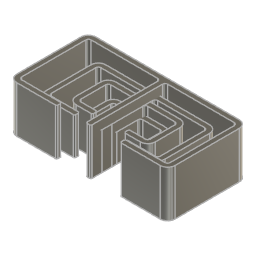
cable clip (Autodesk Fusion 360 design; units mm, degrees)
Autodesk Fusion 360 part; units mm, degrees
other "Base Mesh Feature1"
sketch "Sketch1" plane through (0, 0, 0) normal (0, 0, 1) x (1, 0, 0) in component "Clip-medium"
  line L0 (13, 8) -> (-13, 8)
  line L1 (-16, 5) -> (-16, -5)
  line L2 (16, -5) -> (16, 5)
  line L3 (16, 8) -> (-16, -8) construction
  line L4 (-16, 8) -> (16, -8) construction
  line L5 (-6.4, -8) -> (6.4, -8) construction
  line L6 (6.4, -8) -> (6.4, -6)
  line L7 (6.4, -6) -> (-6.4, -6) construction
  line L8 (-6.4, -6) -> (-6.4, -8)
  arc A0 (-13, 8) -> (-16, 5) centre (-13, 5) ccw
  arc A1 (16, 5) -> (13, 8) centre (13, 5) ccw
  arc A2 (13, -8) -> (16, -5) centre (13, -5) ccw
  arc A3 (-16, -5) -> (-13, -8) centre (-13, -5) ccw
  line L9 (-13, -8) -> (-6.4, -8)
  line L10 (6.4, -8) -> (13, -8)
  line L11 (6.4, -6) -> (13, -6)
  arc A4 (13, -6) -> (14, -5) centre (13, -5) ccw
  line L12 (14, -5) -> (14, 5)
  arc A5 (14, 5) -> (13, 6) centre (13, 5) ccw
  arc A6 (-13, 6) -> (-14, 5) centre (-13, 5) ccw
  line L13 (-14, 5) -> (-14, -5)
  arc A7 (-14, -5) -> (-13, -6) centre (-13, -5) ccw
  line L14 (-13, -6) -> (-6.4, -6)
  line L15 (0, 1.75) -> (0, 22.5) construction
  line L16 (-1, -8) -> (1, -8)
  line L17 (1, -8) -> (1, 6)
  line L18 (-1, 6) -> (-1, -8)
  line L19 (13, 6) -> (1, 6)
  line L20 (-1, 6) -> (-13, 6)
  dimension "d21" = 32
  dimension "d22" = 16
  dimension "d24" = 3
  dimension "d25" = 3
  dimension "d26" = 3
  dimension "d27" = 3
  dimension "d29" = 12.8
  dimension "d30" = 2
  constraint horizontal L0
  constraint perpendicular L0 L1
  constraint parallel L0 L9
  constraint parallel L1 L2
  constraint coincident L3 origin
  constraint coincident L4 origin
  constraint horizontal L5
  constraint vertical L6
  constraint horizontal L7
  constraint vertical L8
  constraint coincident L4.start L1
  constraint coincident L4.start L0
  constraint tangent L1 A0
  constraint tangent L0 A0
  constraint coincident L3.start L0
  constraint coincident L3.start L2
  constraint tangent L0 A1
  constraint tangent L2 A1
  constraint coincident L4.end L2
  constraint coincident L4.end L9
  constraint tangent L2 A2
  constraint tangent A2 L9
  constraint coincident L3.end L1
  constraint coincident L3.end L9
  constraint tangent L1 A3
  constraint tangent A3 L9
  constraint collinear L9 L10
  constraint horizontal L16
  constraint vertical L17
  constraint vertical L18
  constraint coincident L5 L16.start
  constraint concentric A2 A4
  constraint concentric A1 A5
  constraint concentric A0 A6
  constraint concentric A3 A7
  constraint tangent L13 A7
  constraint tangent A5 L19
  constraint tangent A4 L12
  constraint tangent L12 A5
  constraint tangent A6 L19
  constraint tangent A6 L13
  constraint collinear L19 L20
  constraint coincident L7.end L8.start
  measures "d21" distance of L3.end L4.end
  measures "d22" distance of L4.start L3.end
  measures "d24" radius of A0
  measures "d25" radius of A1
  measures "d26" radius of A2
  measures "d27" radius of A3
  measures "d29" distance of L7.end L6.end
  measures "d30" distance of L16.start L16.end
extrude "Extrude1" add sketch "Sketch1" along normal blind 15 makes body 1 in component "Clip-medium"
fillet "Fillet1" radius 0.5 6 edges at (-6.4, -8, 7.5) (-6.4, -6, 7.5) (-1, -8, 7.5) (1, -8, 7.5) (6.4, -8, 7.5) (6.4, -6, 7.5) on bodies 1 in component "Clip-medium"
fillet "Fillet1'" radius 1 2 edges at (-1, 6, 7.5) (1, 6, 7.5) on bodies 1 in component "Clip-medium"
sketch "Sketch1 (2)" plane through (0, 0, 0) normal (0, 0, 1) x (1, 0, 0) in component "Clip-small"
  line L0 (9, 6) -> (-9, 6)
  line L1 (-12, 3) -> (-12, -3)
  line L2 (12, -3) -> (12, 3)
  line L3 (12, 6) -> (-12, -6) construction
  line L4 (-12, 6) -> (12, -6) construction
  line L5 (-4.8, -6) -> (4.8, -6) construction
  line L6 (4.8, -6) -> (4.8, -4)
  line L7 (4.8, -4) -> (-4.8, -4) construction
  line L8 (-4.8, -4) -> (-4.8, -6)
  arc A0 (-9, 6) -> (-12, 3) centre (-9, 3) ccw
  arc A1 (12, 3) -> (9, 6) centre (9, 3) ccw
  arc A2 (9, -6) -> (12, -3) centre (9, -3) ccw
  arc A3 (-12, -3) -> (-9, -6) centre (-9, -3) ccw
  line L9 (-9, -6) -> (-4.8, -6)
  line L10 (4.8, -6) -> (9, -6)
  line L11 (4.8, -4) -> (9, -4)
  arc A4 (9, -4) -> (10, -3) centre (9, -3) ccw
  line L12 (10, -3) -> (10, 3)
  arc A5 (10, 3) -> (9, 4) centre (9, 3) ccw
  arc A6 (-9, 4) -> (-10, 3) centre (-9, 3) ccw
  line L13 (-10, 3) -> (-10, -3)
  arc A7 (-10, -3) -> (-9, -4) centre (-9, -3) ccw
  line L14 (-9, -4) -> (-4.8, -4)
  line L15 (0, 1.75) -> (0, 22.5) construction
  line L16 (-1.0119, -6) -> (0.9881, -6)
  line L17 (0.9881, -6) -> (0.9881, 4)
  line L18 (-1.0119, 4) -> (-1.0119, -6)
  line L19 (9, 4) -> (0.9881, 4)
  line L20 (-1.0119, 4) -> (-9, 4)
  dimension "d21_1" = 24
  dimension "d22_1" = 12
  dimension "d24_1" = 3
  dimension "d25_1" = 3
  dimension "d26_1" = 3
  dimension "d27_1" = 3
  dimension "d29_1" = 9.6
  dimension "d30_1" = 2
  constraint horizontal L0
  constraint perpendicular L0 L1
  constraint parallel L0 L9
  constraint parallel L1 L2
  constraint coincident L3 origin
  constraint coincident L4 origin
  constraint horizontal L5
  constraint vertical L6
  constraint horizontal L7
  constraint vertical L8
  constraint coincident L4.start L1
  constraint coincident L4.start L0
  constraint tangent L1 A0
  constraint tangent L0 A0
  constraint coincident L3.start L0
  constraint coincident L3.start L2
  constraint tangent L0 A1
  constraint tangent L2 A1
  constraint coincident L4.end L2
  constraint coincident L4.end L9
  constraint tangent L2 A2
  constraint tangent A2 L9
  constraint coincident L3.end L1
  constraint coincident L3.end L9
  constraint tangent L1 A3
  constraint tangent A3 L9
  constraint collinear L9 L10
  constraint horizontal L16
  constraint vertical L17
  constraint vertical L18
  constraint coincident L5 L16.start
  constraint concentric A2 A4
  constraint concentric A1 A5
  constraint concentric A0 A6
  constraint concentric A3 A7
  constraint tangent L13 A7
  constraint tangent A5 L19
  constraint tangent A4 L12
  constraint tangent L12 A5
  constraint tangent A6 L19
  constraint tangent A6 L13
  constraint collinear L19 L20
  constraint coincident L7.end L8.start
  measures "d21_1" distance of L3.end L4.end
  measures "d22_1" distance of L4.start L3.end
  measures "d24_1" radius of A0
  measures "d25_1" radius of A1
  measures "d26_1" radius of A2
  measures "d27_1" radius of A3
  measures "d29_1" distance of L7.end L6.end
  measures "d30_1" distance of L16.start L16.end
extrude "Extrude1'" add sketch "Sketch1 (2)" along normal blind 11.25 separate body makes body 2 in component "Clip-small"
fillet "Fillet1''" radius 0.5 6 edges at (-4.8, -6, 5.625) (-4.8, -4, 5.625) (-1.0119, -6, 5.625) (0.9881, -6, 5.625) (4.8, -6, 5.625) (4.8, -4, 5.625) on bodies 2 in component "Clip-small"
fillet "Fillet1'''" radius 1 2 edges at (-1.0119, 4, 5.625) (0.9881, 4, 5.625) on bodies 2 in component "Clip-small"
sketch "Sketch1 (3)" plane through (0, 0, 0) normal (0, 0, 1) x (1, 0, 0) in component "Clip-large"
  line L0 (21, 12) -> (-21, 12)
  line L1 (-24, 9) -> (-24, -9)
  line L2 (24, -9) -> (24, 9)
  line L3 (24, 12) -> (-24, -12) construction
  line L4 (-24, 12) -> (24, -12) construction
  line L5 (-9.6, -12) -> (9.6, -12) construction
  line L6 (9.6, -12) -> (9.6, -10)
  line L7 (9.6, -10) -> (-9.6, -10) construction
  line L8 (-9.6, -10) -> (-9.6, -12)
  arc A0 (-21, 12) -> (-24, 9) centre (-21, 9) ccw
  arc A1 (24, 9) -> (21, 12) centre (21, 9) ccw
  arc A2 (21, -12) -> (24, -9) centre (21, -9) ccw
  arc A3 (-24, -9) -> (-21, -12) centre (-21, -9) ccw
  line L9 (-21, -12) -> (-9.6, -12)
  line L10 (9.6, -12) -> (21, -12)
  line L11 (9.6, -10) -> (20.9991, -10)
  arc A4 (20.9991, -10) -> (22, -9) centre (21, -9) ccw
  line L12 (22, -9) -> (22, 9)
  arc A5 (22, 9) -> (21, 10) centre (21, 9) ccw
  arc A6 (-21, 10) -> (-22, 9) centre (-21, 9) ccw
  line L13 (-22, 9) -> (-22, -9)
  arc A7 (-22, -9) -> (-21, -10) centre (-21, -9) ccw
  line L14 (-21, -10) -> (-9.6, -10)
  line L15 (0, 1.75) -> (0, 22.5) construction
  line L16 (-1.0024, -12) -> (0.9976, -12)
  line L17 (0.9976, -12) -> (0.9976, 10)
  line L18 (-1.0024, 10) -> (-1.0024, -12)
  line L19 (21, 10) -> (0.9976, 10)
  line L20 (-1.0024, 10) -> (-21, 10)
  dimension "d21_2" = 48
  dimension "d22_2" = 24
  dimension "d24_2" = 3
  dimension "d25_2" = 3
  dimension "d26_2" = 3
  dimension "d27_2" = 3
  dimension "d29_2" = 19.2
  dimension "d30_2" = 2
  constraint horizontal L0
  constraint perpendicular L0 L1
  constraint parallel L0 L9
  constraint parallel L1 L2
  constraint coincident L3 origin
  constraint coincident L4 origin
  constraint horizontal L5
  constraint vertical L6
  constraint horizontal L7
  constraint vertical L8
  constraint coincident L4.start L1
  constraint coincident L4.start L0
  constraint tangent L1 A0
  constraint tangent L0 A0
  constraint coincident L3.start L0
  constraint coincident L3.start L2
  constraint tangent L0 A1
  constraint tangent L2 A1
  constraint coincident L4.end L2
  constraint coincident L4.end L9
  constraint tangent L2 A2
  constraint tangent A2 L9
  constraint coincident L3.end L1
  constraint coincident L3.end L9
  constraint tangent L1 A3
  constraint tangent A3 L9
  constraint collinear L9 L10
  constraint horizontal L16
  constraint vertical L17
  constraint vertical L18
  constraint coincident L5 L16.start
  constraint concentric A2 A4
  constraint concentric A1 A5
  constraint concentric A0 A6
  constraint concentric A3 A7
  constraint tangent L13 A7
  constraint tangent A5 L19
  constraint tangent A4 L12
  constraint tangent L12 A5
  constraint tangent A6 L19
  constraint tangent A6 L13
  constraint collinear L19 L20
  constraint coincident L7.end L8.start
  measures "d21_2" distance of L3.end L4.end
  measures "d22_2" distance of L4.start L3.end
  measures "d24_2" radius of A0
  measures "d25_2" radius of A1
  measures "d26_2" radius of A2
  measures "d27_2" radius of A3
  measures "d29_2" distance of L7.end L6.end
  measures "d30_2" distance of L16.start L16.end
extrude "Extrude1''" add sketch "Sketch1 (3)" along normal blind 15 separate body makes body 3 in component "Clip-large"
fillet "Fillet1''''" radius 0.5 6 edges at (-9.6, -12, 7.5) (-9.6, -10, 7.5) (-1.0024, -12, 7.5) (0.9976, -12, 7.5) (9.6, -12, 7.5) (9.6, -10, 7.5) on bodies 3 in component "Clip-large"
fillet "Fillet1'''''" radius 1 2 edges at (-1.0024, 10, 7.5) (0.9976, 10, 7.5) on bodies 3 in component "Clip-large"
sketch "Sketch1 (4)" plane through (0, 0, 0) normal (0, 0, 1) x (1, 0, 0) in component "Clip-XL"
  line L0 (29, 16) -> (-29, 16)
  line L1 (-32, 13) -> (-32, -13)
  line L2 (32, -13) -> (32, 13)
  line L3 (32, 16) -> (-32, -16) construction
  line L4 (-32, 16) -> (32, -16) construction
  line L5 (-12.8, -16) -> (12.8, -16) construction
  line L6 (12.8, -16) -> (12.8, -14)
  line L7 (12.8, -14) -> (-12.8, -14) construction
  line L8 (-12.8, -14) -> (-12.8, -16)
  arc A0 (-29, 16) -> (-32, 13) centre (-29, 13) ccw
  arc A1 (32, 13) -> (29, 16) centre (29, 13) ccw
  arc A2 (29, -16) -> (32, -13) centre (29, -13) ccw
  arc A3 (-32, -13) -> (-29, -16) centre (-29, -13) ccw
  line L9 (-29, -16) -> (-12.8, -16)
  line L10 (12.8, -16) -> (29, -16)
  line L11 (12.8, -14) -> (29.0009, -14)
  arc A4 (29.0009, -14) -> (30, -13) centre (29, -13) ccw
  line L12 (30, -13) -> (30, 13)
  arc A5 (30, 13) -> (29, 14) centre (29, 13) ccw
  arc A6 (-29, 14) -> (-30, 13) centre (-29, 13) ccw
  line L13 (-30, 13) -> (-30, -13)
  arc A7 (-30, -13) -> (-29, -14) centre (-29, -13) ccw
  line L14 (-29, -14) -> (-12.8, -14)
  line L15 (0, 1.75) -> (0, 22.5) construction
  line L16 (-1.0038, -16) -> (0.9962, -16)
  line L17 (0.9962, -16) -> (0.9962, 14)
  line L18 (-1.0038, 14) -> (-1.0038, -16)
  line L19 (29, 14) -> (0.9962, 14)
  line L20 (-1.0038, 14) -> (-29, 14)
  dimension "d21_3" = 64
  dimension "d22_3" = 32
  dimension "d24_3" = 3
  dimension "d25_3" = 3
  dimension "d26_3" = 3
  dimension "d27_3" = 3
  dimension "d29_3" = 25.6
  dimension "d30_3" = 2
  constraint horizontal L0
  constraint perpendicular L0 L1
  constraint parallel L0 L9
  constraint parallel L1 L2
  constraint coincident L3 origin
  constraint coincident L4 origin
  constraint horizontal L5
  constraint vertical L6
  constraint horizontal L7
  constraint vertical L8
  constraint coincident L4.start L1
  constraint coincident L4.start L0
  constraint tangent L1 A0
  constraint tangent L0 A0
  constraint coincident L3.start L0
  constraint coincident L3.start L2
  constraint tangent L0 A1
  constraint tangent L2 A1
  constraint coincident L4.end L2
  constraint coincident L4.end L9
  constraint tangent L2 A2
  constraint tangent A2 L9
  constraint coincident L3.end L1
  constraint coincident L3.end L9
  constraint tangent L1 A3
  constraint tangent A3 L9
  constraint collinear L9 L10
  constraint horizontal L16
  constraint vertical L17
  constraint vertical L18
  constraint coincident L5 L16.start
  constraint concentric A2 A4
  constraint concentric A1 A5
  constraint concentric A0 A6
  constraint concentric A3 A7
  constraint tangent L13 A7
  constraint tangent A5 L19
  constraint tangent A4 L12
  constraint tangent L12 A5
  constraint tangent A6 L19
  constraint tangent A6 L13
  constraint collinear L19 L20
  constraint coincident L7.end L8.start
  measures "d21_3" distance of L3.end L4.end
  measures "d22_3" distance of L4.start L3.end
  measures "d24_3" radius of A0
  measures "d25_3" radius of A1
  measures "d26_3" radius of A2
  measures "d27_3" radius of A3
  measures "d29_3" distance of L7.end L6.end
  measures "d30_3" distance of L16.start L16.end
extrude "Extrude1'''" add sketch "Sketch1 (4)" along normal blind 18.75 separate body makes body 4 in component "Clip-XL"
fillet "Fillet1''''''" radius 0.5 6 edges at (-12.8, -16, 9.375) (-12.8, -14, 9.375) (-1.0038, -16, 9.375) (0.9962, -16, 9.375) (12.8, -16, 9.375) (12.8, -14, 9.375) on bodies 4 in component "Clip-XL"
fillet "Fillet1'''''''" radius 1 2 edges at (-1.0038, 14, 9.375) (0.9962, 14, 9.375) on bodies 4 in component "Clip-XL"
component "Clip-medium" placed x (1, 0, 0) y (0, 1, 0) z (0, 0, 1) at (0, 0, 0)
component "Clip-small" placed x (1, 0, 0) y (0, 1, 0) z (0, 0, 1) at (0, 0, 0)
component "Clip-large" placed x (1, 0, 0) y (0, 1, 0) z (0, 0, 1) at (0, 0, 0)
component "Clip-XL" placed x (1, 0, 0) y (0, 1, 0) z (0, 0, 1) at (0, 0, 0)
equation "thickness = 2 mm"
equation "width = 16 mm"
equation "length = 32 mm"
equation "height = 15 mm"
equation "filletRadius = thickness * 1.5"
equation "d17 = height"
equation "d21 = length"
equation "d22 = width"
equation "opening = 0.4 * length"
equation "d24 = filletRadius"
equation "d25 = filletRadius"
equation "d29 = opening"
equation "d32 = thickness / 4"
equation "d17_1 = height * smallScale"
equation "d21_1 = length * smallScale"
equation "d22_1 = width * smallScale"
equation "d24_1 = filletRadius"
equation "d25_1 = filletRadius"
equation "d29_1 = opening * smallScale"
equation "d32_1 = thickness / 4"
equation "smallScale = 0.75"
equation "d17_2 = height"
equation "d21_2 = length * largeScale"
equation "d22_2 = width * largeScale"
equation "d24_2 = filletRadius"
equation "d25_2 = filletRadius"
equation "d29_2 = opening * largeScale"
equation "d32_2 = thickness / 4"
equation "largeScale = 1.5"
equation "xlScale = 2"
equation "d17_3 = height * 1.25"
equation "d21_3 = length * xlScale"
equation "d22_3 = width * xlScale"
equation "d24_3 = filletRadius"
equation "d25_3 = filletRadius"
equation "d29_3 = opening * xlScale"
equation "d32_3 = thickness / 4"
equation "d37 = filletRadius - thickness"
equation "d39 = filletRadius - thickness"
equation "d41 = filletRadius - thickness"
equation "d43 = filletRadius - thickness"
named bodies: "medium"
